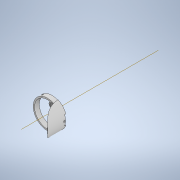
# Autodesk Inventor part: Deckel_Parachute_6
Saved by Autodesk Inventor 2020 (Build 240168000, 168)
## iProperties
Created: 2022-01-25
Part Number: Deckel_Parachute_6
Material: Generisch
Document SubType Name: Modeling
Designer: sp
Density: 1 g/cm^3
Appearance: Vorgabe
Author: sp
## iProperties of the stored document _3D-Druck.ipt
Created: 2022-05-02
Part Number: _3D-Druck
Material: Generisch
Document SubType Name: Modeling
Designer: sp
Density: 1 g/cm^3
Appearance: Vorgabe
Author: sp
Autodesk Inventor part; units mm, degrees
sketch "Skizze1" plane through (0, 0, 0) normal (0, 0, 1) x (1, 0, 0)
  circle A0 centre (0, 0) radius 31
  circle A1 centre (0, 0) radius 29
  dimension "d0" = 62
  dimension "d1" = 58
  constraints: 2 centre point, 2 coincident
  measures "d0" diameter of A0
  measures "d1" diameter of A1
extrude "Extrusion1" add sketch "Skizze1" along normal mid plane 300
sketch "Skizze2" plane through (0, 0, 0) normal (0, 1, 0) x (-1, 0, 0)
  line L0 (-11, 169.5773) -> (-11, -169.8146) construction
  line L1 (-74.8376, 0) -> (82.6362, 0) construction
  line L2 (-11, 75) -> (-11, -75)
  line L3 (-31, -150) -> (-31, 150) projected
  line L4 (31, 150) -> (-31, 150) projected
  line L5 (-31, -150) -> (31, -150) projected
  spline S0 degree 2 poles (-11, 75) (-17.8298, 136.4739) (-72.8449, 128.3193) knots 0 0 0 1 1 1
  spline S1 degree 2 poles (-11, -75) (-17.6171, -136.2673) (-74.8376, -130) knots 0 0 0 1 1 1
  line L6 (-72.8449, 128.3193) -> (-74.8376, -130)
  line L7 (-31, 120) -> (-31, 150)
  line L8 (-31, 150) -> (31, 150)
  line L9 (31, 150) -> (31, -150)
  line L10 (31, -150) -> (31, 150) projected
  line L11 (31, -150) -> (-31, -150)
  line L12 (-31, -150) -> (-31, -120)
  point P0 (0, 0)
  dimension "d4" = 11
  dimension "d5" = 150
  dimension "d6" = 30
  dimension "d7" = 30
  constraints: 18 end point, 5 point on line, 3 perpendicular, 2 collinear, 1 horizontal, 1 symmetric about line, 1 vertical, 6 other
  measures "d4" distance from line of point (0, 0) L0
  measures "d5" distance of L2.start L2.end
  measures "d6" distance from line of L7.start L4
  measures "d7" distance from line of L12.end L5
extrude "Extrusion3" cut sketch "Skizze2" along normal mid plane 100 contours S0 L3 L4 L9 L5 S1 L2
ref_plane "Arbeitsebene3" through (0, 33.25, 0) normal (0, 1, 0) x (-1, 0, 0)
sketch "Skizze8" plane through (0, 33.25, 0) normal (0, 1, 0) x (-1, 0, 0)
  line L0 (-11, -75) -> (-11, 75) projected
  arc A0 (-11, 56.4646) -> (-14.2842, 92.4804) centre (-300.1138, 48.2584) ccw
  arc A1 (-11, 56.4646) -> (-14.2842, 92.4804) centre (-31.6354, 72.7405) ccw
  point P0 (0, 0)
  constraints: 4 point on circle, 2 centre point, 1 point on line
extrude "Extrusion6" cut sketch "Skizze8" against normal blind 65
mirror "Spiegeln2" about plane through (0, 0, 0) normal (0, 0, 1) of "Extrusion6"
ref_plane "Arbeitsebene7" through (15, 0, 0) normal (1, 0, 0) x (0, 1, 0)
sketch "Skizze16" plane through (15, 0, 0) normal (1, 0, 0) x (0, 1, 0)
  line L0 (58.1108, 80) -> (-63.908, 80) construction
  line L1 (50.2709, 80) -> (-47.478, 80)
  line L2 (-47.478, 80) -> (-47.478, -133.5586)
  line L3 (-47.478, -133.5586) -> (50.2709, -133.5586)
  line L4 (50.2709, -133.5586) -> (50.2709, 80)
  point P0 (0, 0)
  point P1 (0, 120)
  dimension "d83" = 40
  constraints: 10 end point, 2 horizontal, 2 parallel, 1 perpendicular, 1 point on line
  measures "d83" distance from line of point (0, 120) L0
extrude "Extrusion15" cut sketch "Skizze16" along normal mid plane 35
ref_plane "Arbeitsebene8" through (0, 0, 80) normal (0, 0, 1) x (1, 0, 0)
sketch "Skizze17" plane through (0, 0, 80) normal (0, 0, 1) x (1, 0, 0)
  circle A0 centre (0, 0) radius 30
  circle A1 centre (0, 0) radius 27
  circle A2 centre (10, -22) radius 4.15
  circle A3 centre (10, 22) radius 4.15
  line L0 (0, -71.2337) -> (0, 71.2337) construction
  line L1 (10, -73.8359) -> (10, 73.0552) construction
  line L2 (44.4276, 0) -> (-43.7851, 0) construction
  circle A4 centre (10, -22) radius 5
  circle A5 centre (10, 22) radius 5
  circle A6 centre (10, -22) radius 6.5
  circle A7 centre (10, 22) radius 6.5
  point P0 (5.2878, 26.4772)
  point P1 (16.4716, 21.3936)
  point P2 (14.0062, 23.083)
  point P3 (8.1818, 25.7305)
  point P4 (16.4716, -21.3936)
  point P5 (5.2878, -26.4772)
  point P6 (8.1818, -25.7305)
  point P7 (14.0062, -23.083)
  dimension "d87" = 54
  dimension "d88" = 10
  dimension "d89" = 44
  dimension "d90" = 8.3
  dimension "d91" = 8.3
  dimension "d92" = 10
  dimension "d93" = 10
  dimension "d96" = 13
  dimension "d97" = 13
  dimension "d127" = 60
  constraints: 8 centre point, 6 coincident, 6 end point, 4 point on line, 2 midpoint, 2 vertical, 1 horizontal, 1 symmetric about line
  measures "d87" diameter of A1
  measures "d88" distance between parallel lines of L0 L1
  measures "d89" distance of A3.centre A2.centre
  measures "d90" diameter of A3
  measures "d91" diameter of A2
  measures "d92" diameter of A4
  measures "d93" diameter of A5
  measures "d96" diameter of A6
  measures "d97" diameter of A7
  measures "d127" diameter of A0
extrude "Extrusion16" add sketch "Skizze17" along normal blind 10 contours A0 A6 A1 A7 | A7 A1 A5 A0 | A0 A6 A1 A4 | A7 A1 A6 A0 | A5 A1 A3 | A1 A2 A4 | A3 A1 | A1 A2 picked at (8.7837, 26.5328) picked at (8.7837, -26.5328) picked at (11.3484, 24.9664) picked at (11.3484, -24.9664)
extrude "Extrusion17" add sketch "Skizze17" along normal blind 10 contours A1 A5 A7 | A6 A1 A4 | A1 A3 A5 | A4 A1 A2 picked at (14.6302, 21.2788) picked at (14.6302, -21.2788)
extrude "Extrusion18" cut sketch "Skizze17" along normal blind 10 contours A3 A1 | A1 A2 picked at (11.3484, 24.9664) picked at (11.3484, -24.9664)
ref_plane "Arbeitsebene9" through (27.75, 0, 0) normal (1, 0, 0) x (0, 1, 0)
sketch "Skizze18" plane through (27.75, 0, 0) normal (1, 0, 0) x (0, 1, 0)
  line L0 (0, 67.103) -> (0, 101.1615) construction
  line L1 (30, 80) -> (-30, 80) construction
  line L2 (-11, 80) -> (11, 80)
  line L3 (11, 80) -> (11, 92)
  line L4 (11, 92) -> (-11, 92)
  line L5 (-11, 92) -> (-11, 80)
  point P0 (0, 0)
  point P1 (0, 80)
  point P2 (27.2115, 80)
  point P3 (-27.2115, 80)
  dimension "d103" = 22
  dimension "d104" = 12
  constraints: 10 end point, 2 parallel, 2 point on line, 1 horizontal, 1 midpoint, 1 perpendicular, 1 vertical, 1 other
  measures "d103" distance of L4.end L3.end
  measures "d104" distance of L3.end L2.end
extrude "Extrusion19" add sketch "Skizze18" against normal blind 3
sketch "Skizze19" plane through (27.75, 0, 0) normal (1, 0, 0) x (0, 1, 0)
  line L0 (0, 67.088) -> (0, 108.0121) construction
  line L1 (30, 80) -> (-30, 80) projected
  line L2 (-27, 80) -> (27, 80) projected
  line L3 (10.5, 80) -> (-10.5, 80)
  line L4 (-10.5, 80) -> (-10.5, 82)
  line L5 (-10.5, 82) -> (10.5, 82)
  line L6 (10.5, 82) -> (10.5, 80)
  point P0 (0, 0)
  point P1 (0, 80)
  point P2 (27.2115, 80)
  point P3 (-27.2115, 80)
  point P4 (-26.4772, 80)
  point P5 (26.4772, 80)
  dimension "d107" = 21
  dimension "d108" = 2
  constraints: 10 end point, 2 parallel, 2 point on line, 1 horizontal, 1 perpendicular, 1 vertical, 3 other
  measures "d107" distance of L4.end L5.end
  measures "d108" distance of L3.end L4.end
extrude "Extrusion20" cut sketch "Skizze19" against normal blind 3
sketch "Skizze20" plane through (27.75, 0, 0) normal (1, 0, 0) x (0, 1, 0)
  circle A0 centre (0, 85) radius 1.75
  line L0 (28.3102, 80) -> (-28.3102, 80) projected
  point P0 (0, 0)
  dimension "d111" = 3.5
  dimension "d112" = 5
  constraints: 1 centre point
  measures "d111" diameter of A0
  measures "d112" distance from line of L0 A0.centre
extrude "Extrusion22" cut sketch "Skizze20" along normal blind 8
pattern_circular "Runde Anordnung2" count 3 over 360 about axis through (0, 0, -10) along (0, 0, 1) of "Extrusion22"
sketch "Skizze21" plane through (0, 0, 80) normal (0, 0, -1) x (-1, 0, 0)
  line L0 (-27.75, 10.5) -> (-24.75, 10.5) projected
  line L1 (-26.75, 10.5) -> (-27.75, 10.5)
  line L2 (-27.75, 10.5) -> (-27.75, -10.5)
  line L3 (-27.75, -10.5) -> (-26.75, -10.5)
  line L4 (-26.75, -10.5) -> (-26.75, 10.5)
  line L5 (-24.75, 10.5) -> (-24.75, -10.5) projected
  point P0 (0, 0)
  dimension "d123" = 1
  dimension "d124" = 2
  constraints: 8 end point, 2 parallel, 1 horizontal, 1 perpendicular, 1 point on line
  measures "d123" distance of L3.end L2.end
  measures "d124" distance between parallel lines of L5 L4
extrude "Extrusion23" cut sketch "Skizze21" against normal blind 10
sketch "Skizze22" plane through (0, 0, 80) normal (0, 0, -1) x (-1, 0, 0)
  line L0 (-27.75, -10.5) -> (-27.75, 10.5) projected
  line L1 (-27.75, -10.5) -> (-31.25, -10.5)
  line L2 (-31.25, -10.5) -> (-31.25, 10.5232)
  line L3 (-31.25, 10.5232) -> (-27.75, 10.5232)
  line L4 (-27.75, 10.5232) -> (-27.75, -10.5)
  point P0 (0, 0)
  dimension "d130" = 3.5
  constraints: 8 end point, 2 parallel, 1 horizontal, 1 perpendicular
  measures "d130" distance of L2.end L3.end
extrude "Extrusion24" cut sketch "Skizze22" against normal blind 2.5
sketch "Skizze23" plane through (15, 0, 0) normal (1, 0, 0) x (0, 1, 0)
  spline S0 degree 3 poles (-26.0905, 99.7877) (-23.9786, 110.207) (-18.6537, 121.4086) (-0.4471, 120.0351) knots 0 0 0 0 1 1 1 1
  spline S1 degree 2 poles (2.7707, 120.0351) (15.3536, 119.9906) (20.3449, 111.9658) knots 0 0 0 1 1 1
  line L0 (-26.0905, 99.7877) -> (-3.4467, 113.8795)
  line L1 (-3.4467, 113.8795) -> (18.4445, 110.2095)
  line L2 (18.4445, 110.2095) -> (20.3449, 111.9658)
  line L3 (2.7707, 120.0351) -> (-0.4471, 120.0351)
  point P0 (0, 0)
  point P1 (-23.0213, 109.094)
  point P2 (-16.4866, 116.6683)
  point P3 (14.154, 117.6561)
  constraints: 8 end point, 1 horizontal, 7 other
extrude "Extrusion25" add sketch "Skizze23" along normal blind 35
ref_plane "Arbeitsebene10" through (0, 0, 121.25) normal (0, 0, 1) x (1, 0, 0)
sketch "Skizze24" plane through (0, 0, 121.25) normal (0, 0, 1) x (1, 0, 0)
  circle A0 centre (0, 0) radius 31
  circle A1 centre (0, 0) radius 29
  circle A2 centre (0, 0) radius 59.5994
  constraints: 3 centre point, 3 coincident
extrude "Extrusion26" cut sketch "Skizze24" against normal blind 30
sketch "Skizze25" plane through (0, 33.25, 0) normal (0, 1, 0) x (-1, 0, 0)
  line L0 (-30.8759, 120.0351) -> (-31, 120.0351) projected
  line L1 (-20.6661, 111.9658) -> (-23.3658, 111.9658) projected
  spline S0 degree 3 poles (-30.8759, 120.0351) (-22.6703, 113.6809) (-15.7283, 100.5324) (-14.0984, 90.712) knots 0 0 0 0 1 1 1 1
  line L2 (-14.0984, 90.712) -> (-7.3509, 98.2926)
  line L3 (-7.3509, 98.2926) -> (-26.0566, 125.5888)
  line L4 (-26.0566, 125.5888) -> (-31, 120.0351)
  point P0 (0, 0)
  point P1 (-30.9968, 120.0351)
  point P2 (-17.1796, 100.871)
  constraints: 6 end point, 1 parallel, 4 other
extrude "Extrusion27" cut sketch "Skizze25" against normal blind 65
